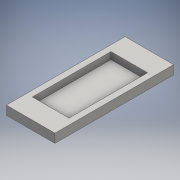
# Autodesk Inventor part: Arduino
Saved by Autodesk Inventor 2016 (Build 200138000, 138)
## iProperties
Created: 2016-04-24
Part Number: Arduino
Material: Generic
Document SubType Name: Modeling
Designer: Freddy Chang
Density: 1 g/cm^3
Appearance: Default
Author: Freddy Chang
Autodesk Inventor part; units mm, degrees
ref_plane "YZ Plane" through (0, 0, 0) normal (1, 0, 0) x (0, 1, 0)
ref_plane "XZ Plane" through (0, 0, 0) normal (0, 1, 0) x (-1, 0, 0)
ref_plane "XY Plane" through (0, 0, 0) normal (0, 0, 1) x (1, 0, 0)
sketch "Sketch1" plane through (0, 0, 0) normal (0, 0, 1) x (1, 0, 0)
  line L0 (0, 0) -> (24.55, 0)
  line L1 (24.55, 0) -> (24.55, -60)
  line L2 (24.55, -60) -> (0, -60)
  line L3 (0, -60) -> (0, 0)
  dimension "d0" = 24.55
  dimension "d1" = 60
  constraints: 8 end point, 2 parallel, 1 horizontal, 1 perpendicular
  measures "d0" distance of L1.end L2.end
  measures "d1" distance of L0.end L1.end
extrude "Extrusion1" add sketch "Sketch1" along normal blind 4.5
sketch "Sketch2" plane through (0, 0, 4.5) normal (0, 0, 1) x (1, 0, 0)
  line L0 (24.55, 0) -> (0, 0) projected
  line L1 (0, -60) -> (24.55, -60) projected
  line L2 (24.55, -60) -> (24.55, 0) projected
  line L3 (21.55, -10.125) -> (21.55, -49.875)
  line L4 (3, -49.875) -> (3, -10.125)
  line L5 (21.55, -30) -> (21.55, -10.125)
  line L6 (21.55, -10.125) -> (3, -10.125)
  line L7 (21.55, -30) -> (21.55, -49.875)
  line L8 (21.55, -49.875) -> (3, -49.875)
  line L9 (0, 0) -> (0, -60) projected
  dimension "d10" = 10.125
  dimension "d11" = 10.125
  dimension "d12" = 3
  dimension "d13" = 3
  constraints: 12 end point, 2 perpendicular, 1 midpoint, 1 parallel
  measures "d10" distance between parallel lines of L0 L6
  measures "d11" distance between parallel lines of L1 L8
  measures "d12" distance between parallel lines of L2 L3
  measures "d13" distance between parallel lines of L9 L4
extrude "Extrusion2" cut sketch "Sketch2" against normal blind 3.5 contours L3 L8 L4 L6
body "Solid1"
